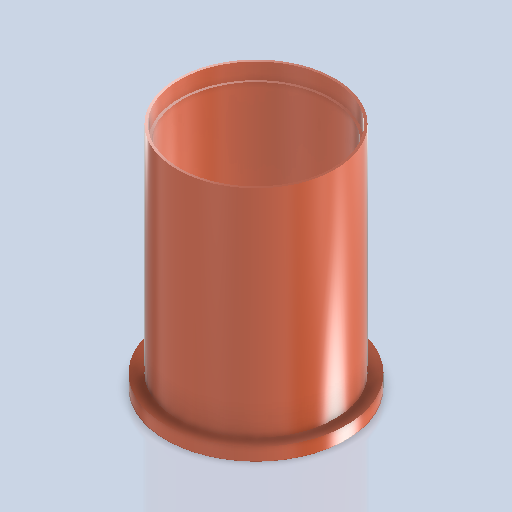
# Autodesk Inventor part: 13
Saved by Autodesk Inventor 2024.2 (Build 282272000, 272)
## iProperties
Created: 2024-05-05
Part Number: 13
Material: Phenolharz
Document SubType Name: Modeling
Designer: Fabri
Density: 1.38 g/cm^3
Appearance: Glatt - Hellorange
Author: Fabri
Autodesk Inventor part; units mm, degrees
ref_plane "YZ Plane" through (0, 0, 0) normal (1, 0, 0) x (0, 1, 0)
ref_plane "XZ Plane" through (0, 0, 0) normal (0, 1, 0) x (-1, 0, 0)
ref_plane "XY Plane" through (0, 0, 0) normal (0, 0, 1) x (1, 0, 0)
sketch "Skizze1" plane through (0, 0, 0) normal (0, 1, 0) x (-1, 0, 0)
  line L0 (0, 0) -> (0, -142)
  line L1 (0, 0) -> (49, 0)
  line L2 (49, 0) -> (49, -134)
  line L3 (49, -134) -> (56, -134)
  line L4 (56, -134) -> (56, -142)
  line L5 (56, -142) -> (0, -142)
  dimension "d0" = 112
  dimension "d1" = 8
  dimension "d2" = 134
  dimension "d3" = 98
  constraints: 12 end point, 4 perpendicular, 1 horizontal, 1 vertical
  measures "d0" diameter of L4 L0
  measures "d1" distance of L3.end L4.end
  measures "d2" distance of L1.end L2.end
  measures "d3" diameter of L2 L0
revolve "Umdrehung1" add sketch "Skizze1" angle 360 about axis through (0, 0, 0) along (0, 0, -1)
sketch "Skizze2" plane through (0, 0, 0) normal (0, 0, 1) x (1, 0, 0)
  circle A0 centre (0, 0) radius 49 projected
  constraints: 1 coincident
hole "Bohrung1" at (0, 0, 0) direction (0, 0, -1) diameter 92 end through all counterbore diameter 95 counterbore depth 10
